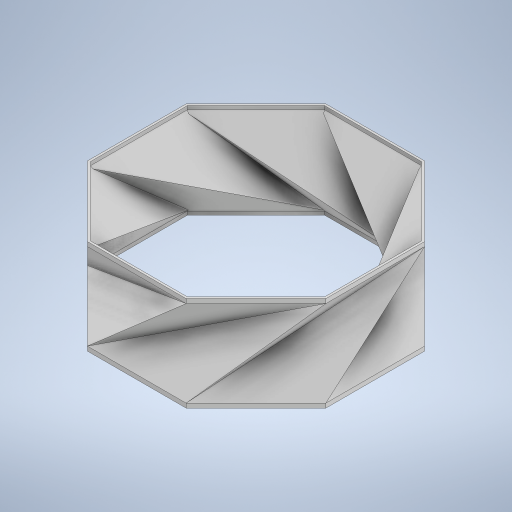
# Autodesk Inventor part: 팔각형 OV-PAM 층 한개
Saved by Autodesk Inventor 2024 (Build 280153000, 153)
## iProperties
Created: 2023-06-16
Part Number: 팔각형 OV-PAM 층 한개
Material: 일반
Document SubType Name: Modeling
Designer: jsw
Density: 1 g/cm^3
Appearance: 기본값
Author: jsw
Autodesk Inventor part; units mm, degrees
ref_plane "YZ Plane" through (0, 0, 0) normal (1, 0, 0) x (0, 1, 0)
ref_plane "XZ Plane" through (0, 0, 0) normal (0, 1, 0) x (-1, 0, 0)
ref_plane "XY Plane" through (0, 0, 0) normal (0, 0, 1) x (1, 0, 0)
sketch "스케치1" plane through (0, 0, 0) normal (0, 1, 0) x (-1, 0, 0)
  line L0 (-32.5919, 13.5) -> (-13.5, 32.5919)
  line L1 (-13.5, 32.5919) -> (13.5, 32.5919)
  line L2 (13.5, 32.5919) -> (32.5919, 13.5)
  line L3 (32.5919, 13.5) -> (32.5919, -13.5)
  line L4 (32.5919, -13.5) -> (13.5, -32.5919)
  line L5 (13.5, -32.5919) -> (-13.5, -32.5919)
  line L6 (-13.5, -32.5919) -> (-32.5919, -13.5)
  line L7 (-32.5919, -13.5) -> (-32.5919, 13.5)
  line L8 (-13.7485, 33.1919) -> (13.7485, 33.1919)
  line L9 (13.7485, 33.1919) -> (33.1919, 13.7485)
  line L10 (33.1919, 13.7485) -> (33.1919, -13.7485)
  line L11 (33.1919, -13.7485) -> (13.7485, -33.1919)
  line L12 (13.7485, -33.1919) -> (-13.7485, -33.1919)
  line L13 (-13.7485, -33.1919) -> (-33.1919, -13.7485)
  line L14 (-33.1919, -13.7485) -> (-33.1919, 13.7485)
  line L15 (-33.1919, 13.7485) -> (-13.7485, 33.1919)
  point P0 (0, 0)
  point P1 (0, 0)
  point P2 (0, 0)
  dimension "d0" = 27
  dimension "d2" = 0.6
  constraints: 32 end point, 2 coincident, 2 horizontal, 34 other
  measures "d0" distance of L0.end L1.end
  measures "d2" distance between parallel lines of L10 L3
extrude "돌출2" add sketch "스케치1" along normal blind 24 contours L0 L1 L2 L3 L4 L5 L6 L7 | L8 L9 L10 L11 L12 L13 L14 L15
ref_plane "작업 평면24" through (-13.7485, 24, -33.1919) normal (0, -0.6294873, -0.7770108) x (1, 0, 0)
sketch "스케치27" plane through (13.7485, 0, -33.1919) normal (0, 0, -1) x (-1, 0, 0)
  line L0 (27.4971, 24) -> (46.9404, 24) projected
  line L1 (0, 24) -> (27.4971, 24) projected
  line L2 (27.4971, 24) -> (0, 24)
  line L3 (0, 24) -> (-19.4434, 0)
  line L4 (-19.4434, 0) -> (27.4971, 24)
  line L5 (0, 0) -> (0, 24) projected
  line L6 (0, 24) -> (0, 9.9411)
  point P0 (13.7485, 0)
  constraints: 8 end point, 2 point on line, 1 horizontal
extrude "돌출22" cut sketch "스케치27" against normal up to surface surface through (-13.7485, 24, -33.1919) normal (0, -0.6294873, -0.7770108)
ref_plane "작업 평면26" through (33.1919, 0, -13.7485) normal (0.5494296, 0.6294873, -0.5494296) x (-0.7071068, 0, -0.7071068)
sketch "스케치28" plane through (13.7485, 0, -33.1919) normal (0.7071068, 0, -0.7071068) x (-0.7071068, 0, -0.7071068)
  line L0 (-27.3314, 0) -> (-27.3314, 12) projected
  line L1 (19.4434, 0) -> (0, 0) projected
  line L2 (-27.4971, 0) -> (0, 0)
  line L3 (19.4434, 0) -> (19.4434, 24) projected
  line L4 (0, 0) -> (19.4434, 24)
  line L5 (19.4434, 24) -> (-27.4971, 0)
  point P0 (-13.7485, 0)
  point P1 (-27.3314, 12)
  constraints: 6 end point, 1 collinear
extrude "돌출23" cut sketch "스케치28" along normal up to surface contours L2 L5 L0 | L0 L5 L4 L2 surface through (33.1919, 0, -13.7485) normal (0.5494296, 0.6294873, -0.5494296)
pattern_circular "원형 패턴5" count 8 over 360 about axis through (0, -10, 0) along (0, 1, 0) of "돌출23", "돌출22"
ref_plane "작업 평면27" through (0, 12, 0) normal (0, 1, 0) x (1, 0, 0)
sketch "스케치31" plane through (0, 24, 0) normal (0, 1, 0) x (1, 0, 0)
  line L0 (33.1919, -13.7485) -> (33.1919, 13.7485) projected
  line L1 (33.1919, 13.7485) -> (13.7485, 33.1919) projected
  line L2 (13.7485, 33.1919) -> (-13.7485, 33.1919) projected
  line L3 (-13.7485, 33.1919) -> (-33.1919, 13.7485) projected
  line L4 (-33.1919, 13.7485) -> (-33.1919, -13.7485) projected
  line L5 (-33.1919, -13.7485) -> (-13.7485, -33.1919) projected
  line L6 (-13.7485, -33.1919) -> (13.7485, -33.1919) projected
  line L7 (13.7485, -33.1919) -> (33.1919, -13.7485) projected
  point P0 (0, 0)
extrude "돌출25" add sketch "스케치31" along normal blind 1.2
mirror "미러10" about plane through (0, 12, 0) normal (0, 1, 0) of "돌출25"
shell "쉘9" thickness 0.6 removed faces 2 at (-1.8983, 25.2, 4.5828) at (-1.8983, -1.2, 4.5828)
